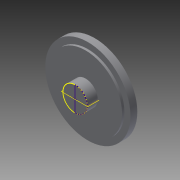
# Autodesk Inventor part: Caps 8mm Square Rounded Caps Male
Saved by Autodesk Inventor 2018 (Build 220112000, 112)
## iProperties
Created: 2017-12-12
Part Number: Caps 8mm Square Rounded Caps Male
Material: Generic
Document SubType Name: Modeling
Designer: Rus
Density: 1 g/cm^3
Appearance: Default
Author: Rus
Autodesk Inventor part; units mm, degrees
ref_plane "YZ Plane" through (0, 0, 0) normal (1, 0, 0) x (0, 1, 0)
ref_plane "XZ Plane" through (0, 0, 0) normal (0, 1, 0) x (-1, 0, 0)
ref_plane "XY Plane" through (0, 0, 0) normal (0, 0, 1) x (1, 0, 0)
sketch "Sketch1" plane through (0, 0, 0) normal (0, 1, 0) x (-1, 0, 0)
  circle A0 centre (0, 0) radius 4
  line L0 (0, 0) -> (4, 0) construction
  line L1 (0, 0) -> (0, -4) construction
  line L2 (0, 0) -> (-4, 0) construction
  line L3 (0, 0) -> (0, 4) construction
  dimension "d0" = 8
  constraints: 8 end point, 4 point on circle, 2 point on line, 1 centre point, 1 coincident, 1 horizontal, 1 perpendicular
  measures "d0" diameter of A0
extrude "Extrusion1" add sketch "Sketch1" against normal blind 3.5
ref_plane "Work Plane1" through (0, 0, 0) normal (0, 0, 1) x (1, 0, 0)
sketch "Sketch2" plane through (0, 0, 0) normal (0, 0, 1) x (1, 0, 0)
  line L0 (-4, 0) -> (4, 0) projected
  line L1 (4, 0) -> (12, 0)
  line L2 (14, 0.75) -> (14, 3)
  line L3 (12.5, 3.75) -> (10.5, 3.75)
  line L4 (0, 0) -> (0, 1.25)
  line L5 (4, 0) -> (4, 1.5959) construction
  line L6 (14, 0.75) -> (12, 0.75)
  line L7 (12, 0.75) -> (12, 0)
  line L8 (14, 3) -> (12.5, 3.75)
  line L9 (10.5, 2.5) -> (10.5, 3.75)
  line L10 (5.8611, 1.9477) -> (6, 1.8384)
  line L11 (6, 1.8384) -> (6.1093, 1.9773)
  line L12 (4.1093, 1.7392) -> (4, 1.6003)
  line L13 (4, 1.6003) -> (3.8611, 1.7097)
  line L14 (1.8611, 1.4716) -> (2, 1.3622)
  line L15 (2, 1.3622) -> (2.1093, 1.5011)
  line L16 (0, 1.25) -> (1.8611, 1.4716)
  line L17 (2.1093, 1.5011) -> (3.8611, 1.7097)
  line L18 (4.1093, 1.7392) -> (5.8611, 1.9477)
  line L19 (4, 1.6003) -> (4, 3.125) construction
  line L20 (6, 1.8384) -> (6, 3.125) construction
  line L21 (10.5, 3.125) -> (6, 3.125) construction
  line L22 (6, 3.125) -> (4, 3.125) construction
  line L23 (4, 3.125) -> (2, 3.125) construction
  line L24 (2, 3.125) -> (0, 3.125) construction
  line L25 (1.8611, 1.4716) -> (2.1093, 1.5011) construction
  line L26 (3.8611, 1.7097) -> (4.1093, 1.7392) construction
  line L27 (5.8611, 1.9477) -> (6.1093, 1.9773) construction
  line L28 (1.9852, 1.4863) -> (2, 1.3622) construction
  line L29 (4, 1.7262) -> (4, 1.6003) construction
  line L30 (2, 1.3622) -> (2, 3.125) construction
  line L31 (7.8611, 2.1858) -> (8, 2.0765)
  line L32 (8, 2.0765) -> (8.1093, 2.2154)
  line L33 (8, 2.0765) -> (8, 3.125) construction
  line L34 (6.1093, 1.9773) -> (7.8611, 2.1858)
  line L35 (8.1093, 2.2154) -> (10.5, 2.5)
  point P0 (6, 1.9643)
  dimension "d8" = 14
  dimension "d11" = 12
  dimension "d12" = 0.75
  dimension "d13" = 3
  dimension "d14" = 0.75
  dimension "d15" = 1.5
  dimension "d16" = 1.25
  dimension "d19" = 3.5
  dimension "d23" = 1.25
  dimension "d24" = 2
  dimension "d25" = 0.125
  dimension "d26" = 2
  dimension "d27" = 2
  constraints: 70 end point, 12 collinear, 11 perpendicular, 8 equal length, 7 point on line, 5 vertical, 4 horizontal, 2 midpoint
  measures "d8" distance between parallel lines of L2 L4
  measures "d11" distance between parallel lines of L7 L4
  measures "d12" distance of L6.end L1.end
  measures "d13" distance between parallel lines of L3 L6
  measures "d14" distance from line of L2.end L3
  measures "d15" distance from line of L2 L3.start
  measures "d16" distance of L4.start L4.end
  measures "d19" horizontal distance of L3.end L2.end
  measures "d23" vertical distance of L4.end L9.start
  measures "d24" distance of L23.end L24.end
  measures "d25" distance of L28.start L14.end
  measures "d26" distance of L19.end L23.end
  measures "d27" distance between parallel lines of L33 L20
revolve "Revolution1" add sketch "Sketch2" angle 360 about axis through (0, 0, 0) along (0, 1, 0)
sketch "Sketch3" plane through (0, -3.5, 0) normal (0, -1, 0) x (1, 0, 0)
  point P0 (0, 0)
  point P1 (0, 0)
  constraints: 1 coincident
sketch "Sketch4" plane through (0, -3.5, 0) normal (0, -1, 0) x (1, 0, 0)
  circle A0 centre (0, 0) radius 4 projected
  circle A1 centre (0, 0) radius 4 projected
  arc A2 (0, -4) -> (0, 4) centre (0, 0) ccw
  line L0 (0, 4) -> (0, -4)
  constraints: 2 end point, 2 point on circle, 2 vertical, 2 vertical alignment, 1 centre point, 1 coincident, 2 other
extrude "Extrusion2" add sketch "Sketch4" along normal blind 2 contours A0 L0 picked at (0.5785, 1.2013)
sketch "Sketch5" plane through (0, -3.5, 0) normal (0, -1, 0) x (1, 0, 0)
  line L0 (0, -4) -> (0, 4) projected
  arc A0 (0, 4) -> (0, -4) centre (0, 0) ccw projected
extrude "Extrusion3" cut sketch "Sketch5" against normal blind 2
body "Solid1"
